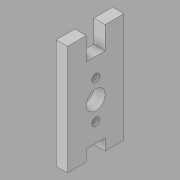
# Autodesk Inventor part: e_support 2
Saved by Autodesk Inventor 2019 (Build 230136000, 136)
## iProperties
Created: 2021-11-02
Part Number: e_support 2
Material: Generic
Document SubType Name: Modeling
Designer: Mohamed
Density: 1 g/cm^3
Appearance: Default
Author: Mohamed
Autodesk Inventor part; units mm, degrees
ref_plane "YZ Plane" through (0, 0, 0) normal (1, 0, 0) x (0, 1, 0)
ref_plane "XZ Plane" through (0, 0, 0) normal (0, 1, 0) x (-1, 0, 0)
ref_plane "XY Plane" through (0, 0, 0) normal (0, 0, 1) x (1, 0, 0)
sketch "Sketch1" plane through (0, 0, 0) normal (1, 0, 0) x (0, 1, 0)
  line L0 (0, 0) -> (40, 0)
  line L1 (40, -10) -> (40, -20)
  line L2 (40, -30) -> (0, -30)
  line L3 (0, -20) -> (0, -10)
  line L4 (40, 0) -> (52, 0)
  line L5 (52, 0) -> (52, -10)
  line L6 (52, -10) -> (40, -10)
  line L7 (40, -30) -> (52, -30)
  line L8 (52, -30) -> (52, -20)
  line L9 (52, -20) -> (40, -20)
  line L10 (0, 0) -> (-6, 0)
  line L11 (-6, 0) -> (-6, -10)
  line L12 (-6, -10) -> (0, -10)
  line L13 (0, -30) -> (-6, -30)
  line L14 (-6, -30) -> (-6, -20)
  line L15 (-6, -20) -> (0, -20)
  circle A0 centre (10, -15) radius 2.1
  circle A1 centre (30, -15) radius 2.1
  circle A2 centre (20, -15) radius 5
  dimension "d0" = 40
  dimension "d1" = 30
  dimension "d2" = 12
  dimension "d3" = 10
  dimension "d4" = 12
  dimension "d5" = 10
  dimension "d6" = 6
  dimension "d7" = 10
  dimension "d8" = 6
  dimension "d9" = 10
  dimension "d12" = 4.2
  dimension "d13" = 4.2
  dimension "d17" = 10
  constraints: 32 end point, 6 parallel, 5 horizontal, 5 perpendicular, 3 centre point
  measures "d0" distance of L2.start L2.end
  measures "d1" distance of L0.end L2.start
  measures "d2" distance of L1.start L5.end
  measures "d3" distance of L4.end L5.end
  measures "d4" distance of L1.end L8.end
  measures "d5" distance of L8.end L7.end
  measures "d6" distance of L3.end L11.end
  measures "d7" distance of L11.end L10.end
  measures "d8" distance of L3.start L14.end
  measures "d9" distance of L13.end L14.end
  measures "d12" diameter of A0
  measures "d13" diameter of A1
  measures "d17" diameter of A2
extrude "Extrusion1" add sketch "Sketch1" along normal blind 6 contours L0 L4 L5 L6 L1 L9 L8 L7 L2 L13 L14 L15 L3 L12 L11 L10 | A2
sketch "Sketch2" plane through (6, 0, 0) normal (1, 0, 0) x (0, 0, -1)
  circle A0 centre (15, 30) radius 2.1 projected
  circle A1 centre (15, 20) radius 5
  point P0 (0, 0)
  dimension "d19" = 10
  constraints: 1 centre point
  measures "d19" diameter of A1
extrude "Extrusion2" cut sketch "Sketch2" against normal blind 6 contours A1
body "Solid1"
